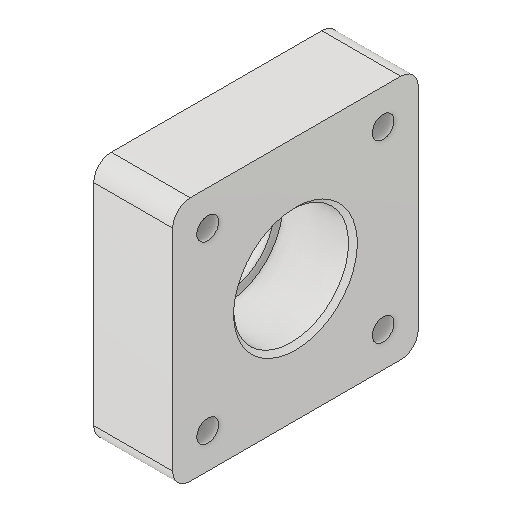
# Autodesk Inventor part: 3DP_PLA_X_axis_idler_bearing_block
Saved by Autodesk Inventor 2026.1 (Build 301233000, 233)
## iProperties
Created: 2018-07-11
Part Number: 3DP_PLA_X_axis_idler_bearing_block
Material: ABS Plastic
Document SubType Name: Modeling
Designer: Andrzej
Density: 1.06 g/cm^3
Appearance: Smooth - White
Author: Andrzej
Autodesk Inventor part; units mm, degrees
ref_plane "YZ Plane" through (0, 0, 0) normal (1, 0, 0) x (0, 1, 0)
ref_plane "XZ Plane" through (0, 0, 0) normal (0, 1, 0) x (-1, 0, 0)
ref_plane "XY Plane" through (0, 0, 0) normal (0, 0, 1) x (1, 0, 0)
sketch "Sketch1" plane through (0, 0, 0) normal (1, 0, 0) x (0, 1, 0)
  line L0 (6.1628, 9.8367) -> (-21.8372, 9.8367)
  line L1 (-21.8372, 9.8367) -> (-21.8372, -18.1633)
  line L2 (-21.8372, -18.1633) -> (6.1628, -18.1633)
  line L3 (6.1628, -18.1633) -> (6.1628, 9.8367)
  circle A0 centre (-7.8372, -4.1633) radius 6.55
  point P0 (0, 0)
  point P1 (2.1628, 5.8367)
  point P2 (-17.8372, 5.8367)
  point P3 (-17.8372, -14.1633)
  point P4 (2.1628, -14.1633)
  dimension "d0" = 28
  dimension "d1" = 28
  dimension "d2" = 20
  dimension "d3" = 20
  dimension "d4" = 4
  dimension "d5" = 4
  dimension "d6" = 14
  dimension "d7" = 14
  dimension "d8" = 13.1
  constraints: 8 end point, 2 horizontal alignment, 2 parallel, 2 vertical alignment, 1 centre point, 1 coincident, 1 horizontal, 1 perpendicular
  measures "d0" distance of L2.end L1.end
  measures "d1" distance of L1.end L0.end
  measures "d2" distance of point (2.163, -14.163) point (2.163, 5.837)
  measures "d3" distance of point (2.163, 5.837) point (-17.837, 5.837)
  measures "d4" distance from line of L3 point (2.163, 5.837)
  measures "d5" distance from line of L0 point (2.163, 5.837)
  measures "d6" distance from line of L3 point (-7.837, -4.163)
  measures "d7" distance from line of L0 point (-7.837, -4.163)
  measures "d8" diameter of A0
extrude "Extrusion1" add sketch "Sketch1" along normal blind 9
hole "Hole1" at (0, 2.1628, 5.8367) at (0, -17.8372, 5.8367) at (0, -17.8372, -14.1633) at (0, 2.1628, -14.1633) direction (1, 0, 0) diameter 2.5 end through all
sketch "Sketch2" plane through (0, 0, 0) normal (-1, 0, 0) x (0, 0, 1)
  circle A0 centre (-14.1633, -17.8372) radius 1.25 projected
  circle A1 centre (5.8367, 2.1628) radius 1.25 projected
  circle A2 centre (5.8367, -17.8372) radius 1.25 projected
  circle A3 centre (-14.1633, 2.1628) radius 1.25 projected
  circle A4 centre (-4.1633, -7.8372) radius 6.55 projected
  line L0 (9.8367, 6.1628) -> (9.8367, -21.8372) projected
  line L1 (-18.1633, 6.1628) -> (9.8367, 6.1628) projected
  line L2 (-18.1633, -21.8372) -> (-18.1633, 6.1628) projected
  line L3 (9.8367, -21.8372) -> (-18.1633, -21.8372) projected
  circle A5 centre (-4.1633, -7.8372) radius 5.55
  point P0 (0, 0)
  dimension "d18" = 1
  constraints: 1 centre point
  measures "d18" radial gap between concentric circles of A4 A5
extrude "Extrusion2" add sketch "Sketch2" against normal blind 1 contours A4
fillet "Fillet1" radius 2 4 edges at (4.5, -21.8372, 9.8367) (4.5, 6.1628, 9.8367) (4.5, -21.8372, -18.1633) (4.5, 6.1628, -18.1633)
chamfer "Chamfer1" distance 0.5 angle 45 1 edges at (9, -14.3872, -4.1633)
body "Solid1"
